Radial Arm Saw Base and Top (Autodesk Fusion 360 design; units mm, degrees)
Autodesk Fusion 360 part; units mm, degrees
note: some values were not read from the file. Chosen so that the rebuilt part matches the saved one: which face or edge a step refers to; where a step ends.
sketch "Sketch1" plane through (0, 0, 0) normal (0, 0, 1) x (1, 0, 0) in component "Base Top"
  line L0 (-234.95, 234.95) -> (234.95, 234.95)
  line L1 (234.95, 234.95) -> (234.95, -234.95)
  line L2 (234.95, -234.95) -> (-234.95, -234.95)
  line L3 (-234.95, -234.95) -> (-234.95, 234.95)
  line L4 (-234.95, 234.95) -> (234.95, -234.95) construction
  line L5 (234.95, 234.95) -> (-234.95, -234.95) construction
  dimension "d1" = 469.9
  dimension "d2" = 469.9
  constraint horizontal L0
  constraint perpendicular L0 L1
  constraint parallel L0 L2
  constraint parallel L1 L3
  constraint coincident L4 origin
  constraint coincident L5 origin
  measures "d1" distance of L1.end L2.end
  measures "d2" distance of L0.end L1.end
extrude "Extrude1" add sketch "Sketch1" along normal blind 19.05 makes body 1 in component "Base Top"
box "BoxPrimitive1" add length 469.9 width 469.9 height 139.7 placed x (0, 1, 0) y (-1, 0, 0) z (0, 0, 1) at (234.95, -234.95, 19.05) separate body makes body 2 in component "Saw Frame"
sketch "Sketch2" plane through (0, -234.95, 0) normal (0, -1, 0) x (1, 0, 0) in component "Saw Frame"
  line L0 (-234.95, 158.75) -> (-234.95, 19.05)
  line L1 (-234.95, 19.05) -> (234.95, 19.05)
  line L2 (234.95, 19.05) -> (234.95, 158.75)
  line L3 (234.95, 158.75) -> (-234.95, 158.75)
  line L4 (-234.95, 158.75) -> (234.95, 158.75)
  line L5 (234.95, 158.75) -> (234.95, 19.05)
  line L6 (234.95, 158.75) -> (260.35, 158.75)
  line L7 (260.35, 158.75) -> (260.35, 155.575)
  line L8 (260.35, 155.575) -> (241.3, 155.575)
  line L9 (238.125, 152.4) -> (238.125, 133.35)
  line L10 (238.125, 133.35) -> (234.95, 133.35)
  arc A0 (238.125, 158.75) -> (234.95, 155.575) centre (238.125, 155.575) ccw
  line L11 (234.95, 155.575) -> (238.125, 155.575) construction
  line L12 (238.125, 155.575) -> (238.125, 158.75) construction
  arc A1 (241.3, 155.575) -> (238.125, 152.4) centre (241.3, 152.4) ccw
  dimension "d18" = 25.4
  dimension "d19" = 25.4
  dimension "d20" = 3.175
  constraint coincident L2.end L3.start
  constraint perpendicular L5 L6
  constraint perpendicular L6 L7
  constraint perpendicular L7 L8
  constraint perpendicular L8 L9
  constraint coincident L2 L10.end
  constraint perpendicular L2 L10
  constraint equal L7 L10
  constraint tangent L5 A0
  constraint coincident L5 A0.end
  constraint coincident L6 A0.start
  constraint tangent L6 A0
  constraint coincident A0.centre L11.end
  constraint tangent L9 A1
  constraint tangent L8 A1
  measures "d18" distance of L2.end L6.end
  measures "d19" distance of L6 L10
  measures "d20" distance of L9.end L10.end
extrude "Extrude1'" add sketch "Sketch2" along normal blind 88.9 and the other way blind 368.3 separate body contours L2 L5 L6 L7 L8 L9 L10 A0 A1 makes body 3 in component "Saw Frame"
sketch "Sketch3" plane through (0, 0, 158.75) normal (0, 0, 1) x (-1, 0, 0) in component "Saw Frame"
  line L0 (-238.125, -133.35) -> (-238.125, 323.85)
  line L1 (-238.125, 323.85) -> (-260.35, 323.85)
  line L2 (-260.35, 323.85) -> (-260.35, -133.35)
  line L3 (-260.35, -133.35) -> (-238.125, -133.35)
  line L4 (-234.95, 323.85) -> (-260.35, 323.85) construction
  line L5 (-247.65, 323.85) -> (-247.65, -273.5996) construction
  circle A0 centre (-247.65, 298.45) radius 7.0708
  circle A1 centre (-247.65, 171.45) radius 7.0708
  line L6 (-252.06, -12.2675) -> (-252.06, -24.4188)
  arc A2 (-252.06, -24.4188) -> (-243.24, -24.4188) centre (-247.65, -24.4188) ccw
  line L7 (-243.24, -24.4188) -> (-243.24, -12.2675)
  arc A3 (-243.24, -12.2675) -> (-252.06, -12.2675) centre (-247.65, -6.35) ccw
  arc A4 (-243.24, -63.0675) -> (-252.06, -63.0675) centre (-247.65, -57.15) ccw
  line L8 (-243.24, -75.2188) -> (-243.24, -63.0675)
  arc A5 (-252.06, -75.2188) -> (-243.24, -75.2188) centre (-247.65, -75.2188) ccw
  line L9 (-252.06, -63.0675) -> (-252.06, -75.2188)
  arc A6 (-243.24, -113.8675) -> (-252.06, -113.8675) centre (-247.65, -107.95) ccw
  line L10 (-243.24, -126.0188) -> (-243.24, -113.8675)
  arc A7 (-252.06, -126.0188) -> (-243.24, -126.0188) centre (-247.65, -126.0188) ccw
  line L11 (-252.06, -113.8675) -> (-252.06, -126.0188)
  point P0 (-234.95, 323.85)
  point P1 (-260.35, 323.85)
  dimension "d21" = 8.8199
  dimension "d23" = 14.76
  dimension "d24" = 29.8587
  dimension "d27" = 0
  dimension "d28" = -50.8
  dimension "d29" = 330.2
  dimension "d30" = 25.4
  dimension "d31" = 152.4
  dimension "d32" = 14.1416
  constraint coincident P0 L4.start
  constraint coincident P1 L1.end
  constraint midpoint L4 L5.start
  constraint perpendicular L4 L5
  constraint coincident L5 A0.centre
  constraint coincident L5 A1.centre
  constraint coincident L5 A3.centre
  constraint tangent L6 A2
  constraint tangent A2 L7
  constraint parallel L6 L7
  constraint coincident L5 A2.centre
  constraint horizontal L6.end A2.end
  constraint equal A0 A1
  measures "d21" distance of L6 L7
  measures "d23" diameter of A3
  measures "d29" distance of L5.start A3.centre
  measures "d30" distance of L5.start A0.centre
  measures "d31" distance of L5.start A1.centre
  measures "d32" diameter of A0
extrude "Extrude2" cut sketch "Sketch3" along normal up to far side of body 3 contours A0 | A1 | L6 A2 L7 A3 | A4 L8 A5 L9 | A6 L10 A7 L11 bodies 3 in component "Saw Frame"
ref_plane "WorkPlane1" through (0, 0, 88.9) normal (1, 0, 0) x (0, 0, -1) in component "Saw Frame"
mirror "Mirror1" about plane through (0, 0, 88.9) normal (1, 0, 0) of bodies 3 makes body 4 in component "Saw Frame"
combine "Combine1" operation add target body 2 tool bodies 4 3 in component "Saw Frame"
ref_plane "WorkPlane1" through (0, 0, -717.55) normal (0, 0, -1) x (-1, 0, 0) in component "Front Left Leg"
sketch "Sketch1 (2)" plane through (0, 0, -717.55) normal (0, 0, -1) x (-1, 0, 0) in component "Front Left Leg"
  line L0 (-234.95, -234.95) -> (234.95, -234.95) construction
  line L1 (234.95, -234.95) -> (234.95, 234.95) construction
  line L2 (234.95, 234.95) -> (-234.95, 234.95) construction
  line L3 (-234.95, 234.95) -> (-234.95, -234.95) construction
  line L4 (355.6, 355.6) -> (-355.6, 355.6) construction
  line L5 (-355.6, 355.6) -> (-355.6, -355.6) construction
  line L6 (-355.6, -355.6) -> (355.6, -355.6) construction
  line L7 (355.6, -355.6) -> (355.6, 355.6) construction
  line L8 (355.6, -355.6) -> (355.6, -374.65) construction
  line L9 (355.6, -355.6) -> (374.65, -355.6) construction
  line L10 (374.65, -374.65) -> (374.65, -228.6) construction
  dimension "d43" = 469.9
  dimension "d44" = 120.65
  dimension "d46" = 19.05
  dimension "d57" = 146.05
  dimension "d58" = 19.05
  constraint perpendicular L6 L8
  constraint perpendicular L7 L9
  constraint equal L8 L9
  constraint vertical L10
  constraint coincident L9.end L10
  measures "d43" distance of L0.start L2.end
  measures "d46" distance of L6.end L9.end
  measures "d57" distance of L10.start L10.end
  measures "d58" distance of L9.end L10.start
ref_plane "WorkPlane2" through (-234.95, -234.95, 19.05) normal (0, -0.98685, 0.161639) x (1, 0, 0) in component "Front Left Leg"
sketch "Sketch2 (2)" plane through (0, -231.8501, 37.9755) normal (0, -0.98685, 0.161639) x (1, 0, 0) in component "Front Left Leg"
  line L0 (-234.95, -19.1776) -> (234.95, -19.1776) construction
  line L1 (355.6, -765.5931) -> (-355.6, -765.5931)
  line L2 (-355.6, -765.5931) -> (-234.95, -19.1776)
  line L3 (-106.3016, -19.1776) -> (-226.9516, -765.5931)
  line L4 (-234.95, -19.1776) -> (-106.3016, -19.1776)
  line L5 (-234.95, -19.1776) -> (-254, -19.1776)
  line L6 (-355.6, -765.5931) -> (-374.65, -765.5931)
  line L7 (-254, -19.1776) -> (-374.65, -765.5931)
  dimension "d45" = 19.05
  dimension "d56" = 127
  constraint coincident L1.end L2.start
  constraint coincident L0.start L2.end
  constraint coincident L0 L3.start
  constraint coincident L1 L3.end
  constraint parallel L1 L6
  constraint coincident L5.end L7.start
  constraint equal L5 L6
  constraint parallel L2 L3
  measures "d45" distance of L0.start L5.end
  measures "d56" distance of L2 L3
sweep "Sweep1" add profiles "Sketch2 (2)" path "Sketch1 (2)" along L8 section 1 contours L1 L2 L3 L4 separate body makes body 5 in component "Front Left Leg"
sweep "Sweep1'" add profiles "Sketch2 (2)" path "Sketch1 (2)" along L10 section 1 contours L2 L5 L6 L7 separate body makes body 6 in component "Left Front Let"
sketch "Sketch2 (3)" plane through (234.95, 0, 0) normal (1, 0, 0) x (0, 1, 0) in component "Base Top"
  line L0 (-234.95, 0) -> (234.95, 0)
  line L1 (234.95, 0) -> (234.95, 19.05)
  line L2 (234.95, 19.05) -> (-234.95, 19.05)
  line L3 (-234.95, 19.05) -> (-234.95, 0)
  line L4 (-234.95, 19.05) -> (-355.6, -717.55)
  line L5 (-234.95, 0) -> (-234.95, 19.05)
  line L6 (-234.95, 0) -> (-238.0703, 0)
  constraint coincident L0.start L3.end
  constraint coincident L4 L6.end
  constraint perpendicular L5 L6
sweep "Sweep1''" add profiles "Sketch2 (3)" along 4 edges at (0, 234.95, 19.05) (-234.95, 0, 19.05) (0, -234.95, 19.05) (234.95, 0, 19.05) section 1 contours L3 L4 L5 L6 on bodies 1 bodies 1 in component "Base Top"
mirror "MirrorComponent1" about plane through (0, 0, 0) normal (0, 0, 1) of bodies 6 makes body 7 in component "Left Front Let(Mirror)"
mirror "MirrorComponent1'" about plane through (0, 0, 0) normal (0, 0, 1) of bodies 5 makes body 8 in component "Front Left Leg(Mirror)"
sketch "Sketch1 (3)" plane through (0, -231.8501, 37.9755) normal (0, 0.98685, -0.161639) x (-1, 0, 0) in component "Front/Rear Brace"
  line L0 (-234.95, -19.1776) -> (-355.6, -765.5931)
  line L1 (-355.6, -765.5931) -> (-226.9516, -765.5931)
  line L2 (-226.9516, -765.5931) -> (-106.3016, -19.1776)
  line L3 (-106.3016, -19.1776) -> (-234.95, -19.1776)
  line L4 (-355.6, -765.5931) -> (-234.95, -19.1776)
  line L5 (355.6, -765.5931) -> (234.95, -19.1776)
  line L6 (-312.2499, -497.4025) -> (312.2499, -497.4025)
  line L7 (-328.6724, -599.0025) -> (328.6724, -599.0025)
  dimension "d71" = 101.6
  constraint coincident L4 L6.start
  constraint coincident L5 L6.end
  constraint horizontal L6
  constraint coincident L4 L7.start
  constraint coincident L5 L7.end
  constraint parallel L6 L7
  measures "d71" distance of L6 L7
extrude "Extrude1''" add sketch "Sketch1 (3)" along normal blind 19.05 separate body contours L0 L2 L4 L6 L7 | L2 L5 L6 L7 makes body 9 in component "Front/Rear Brace"
mirror "MirrorComponent2" about plane through (0, 0, 0) normal (0, 0, 1) of bodies 6 makes body 10 in component "Left Front Let(Mirror) (1)"
mirror "MirrorComponent2'" about plane through (0, 0, 0) normal (0, 0, 1) of bodies 5 makes body 11 in component "Front Left Leg(Mirror) (1)"
mirror "MirrorComponent2''" about plane through (0, 0, 0) normal (0, 0, 1) of bodies 9 makes body 12 in component "Front/Rear Brace(Mirror)"
mirror "MirrorComponent2'''" about plane through (0, 0, 0) normal (0, 0, 1) of bodies 7 makes body 13 in component "Left Front Let(Mirror)(Mirror)"
mirror "MirrorComponent2''''" about plane through (0, 0, 0) normal (0, 0, 1) of bodies 8 makes body 14 in component "Front Left Leg(Mirror)(Mirror)"
sketch "Sketch1 (4)" plane through (-231.8501, 0, 37.9755) normal (0.98685, 0, -0.161639) x (0, 1, 0) in component "Left/Right Side Brace"
  line L0 (-107.95, -19.1776) -> (-254, -19.1776)
  line L1 (-254, -19.1776) -> (-374.65, -765.5931)
  line L2 (-374.65, -765.5931) -> (-228.6, -765.5931)
  line L3 (-228.6, -765.5931) -> (-107.95, -19.1776)
  line L4 (-309.8729, -602.0412) -> (-293.4504, -500.4412)
  line L5 (309.8729, -602.0412) -> (293.4504, -500.4412)
  line L6 (-293.4504, -500.4412) -> (293.4504, -500.4412)
  line L7 (309.8729, -602.0412) -> (-309.8729, -602.0412)
  constraint coincident L4.end L6.start
  constraint coincident L5.end L6.end
  constraint coincident L5.start L7.start
  constraint coincident L4.start L7.end
extrude "Extrude1'''" add sketch "Sketch1 (4)" along normal blind 19.05 separate body contours L3 L5 L6 L7 | L3 L4 L6 L7 makes body 15 in component "Left/Right Side Brace"
mirror "MirrorComponent3" about plane through (0, 0, 0) normal (0, 0, 1) of bodies 15 makes body 16 in component "Left/Right Side Brace(Mirror)"
component "Base Top" placed x (1, 0, 0) y (0, 1, 0) z (0, 0, 1) at (0, 0, 0)
component "Saw Frame" placed x (1, 0, 0) y (0, 1, 0) z (0, 0, 1) at (0, 0, 0)
component "Front Left Leg" placed x (1, 0, 0) y (0, 1, 0) z (0, 0, 1) at (0, 0, 0)
component "Left Front Let" placed x (1, 0, 0) y (0, 1, 0) z (0, 0, 1) at (0, 0, 0)
component "Front Left Leg(Mirror)" placed x (-1, 0, 0) y (0, 1, 0) z (0, 0, -1) at (0, 0, 0)
component "Left Front Let(Mirror)" placed x (-1, 0, 0) y (0, 1, 0) z (0, 0, -1) at (0, 0, 0)
component "Front/Rear Brace" placed x (1, 0, 0) y (0, 1, 0) z (0, 0, 1) at (0, 0, 0)
component "Front Left Leg(Mirror) (1)" placed x (1, 0, 0) y (0, -1, 0) z (0, 0, -1) at (0, 0, 0)
component "Left Front Let(Mirror) (1)" placed x (1, 0, 0) y (0, -1, 0) z (0, 0, -1) at (0, 0, 0)
component "Front Left Leg(Mirror)(Mirror)" placed x (-1, 0, 0) y (0, -1, 0) z (0, 0, 1) at (0, 0, 0)
component "Left Front Let(Mirror)(Mirror)" placed x (-1, 0, 0) y (0, -1, 0) z (0, 0, 1) at (0, 0, 0)
component "Front/Rear Brace(Mirror)" placed x (1, 0, 0) y (0, -1, 0) z (0, 0, -1) at (0, 0, 0)
component "Left/Right Side Brace" placed x (1, 0, 0) y (0, 1, 0) z (0, 0, 1) at (0, 0, 0)
component "Left/Right Side Brace(Mirror)" placed x (-1, 0, 0) y (0, 1, 0) z (0, 0, -1) at (0, 0, 0)
equation "d19 = d18"
equation "TopThickness = 1.5 in"
equation "SawFrameHeight = 5.5 in"
equation "TableHeight = 36 in"
equation "BaseRectangleFootprintLength = 28 in"
equation "d41 = TableHeight - TopThickness - SawFrameHeight - MelamineThickness"
equation "MelamineThickness = 0.75 in"
equation "d44 = ( BaseRectangleFootprintLength - 18.5 in ) / 2"
equation "d45 = MelamineThickness"
equation "d46 = MelamineThickness"
equation "d58 = d46"
equation "d72 = MelamineThickness"
equation "d74 = MelamineThickness"
named bodies: "Base Top", "Saw Frame"
